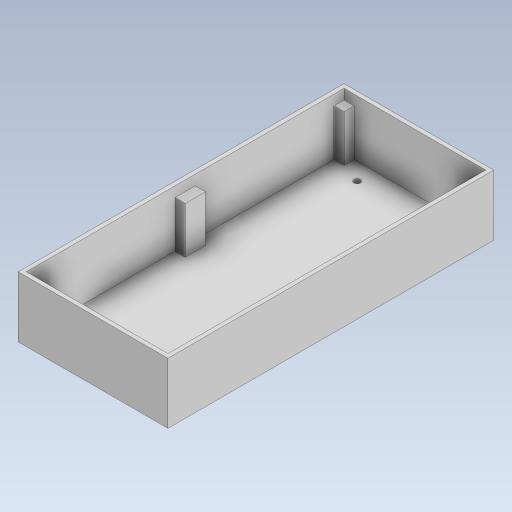
# Autodesk Inventor part: Mounting Master
Saved by Autodesk Inventor 2023.5 (Build 275446000, 446)
## iProperties
Created: 2025-10-29
Part Number: Mounting Master
Material: Generic
Document SubType Name: Modeling
Designer: Guntur
Density: 1 g/cm^3
Appearance: Default
Author: Guntur
## iProperties of the stored document Mounting Master_3DPrint.ipt
Created: 2025-10-29
Part Number: Mounting Master_3DPrint
Material: Generic
Document SubType Name: Modeling
Designer: Guntur
Density: 1 g/cm^3
Appearance: Default
Author: Guntur
Autodesk Inventor part; units mm, degrees
ref_plane "YZ Plane" through (0, 0, 0) normal (1, 0, 0) x (0, 1, 0)
ref_plane "XZ Plane" through (0, 0, 0) normal (0, 1, 0) x (-1, 0, 0)
ref_plane "XY Plane" through (0, 0, 0) normal (0, 0, 1) x (1, 0, 0)
sketch "Sketch1" plane through (0, 0, 0) normal (0, 1, 0) x (-1, 0, 0)
  line L0 (55, 0) -> (-69, 0) construction
  line L1 (0, 72) -> (0, -101) construction
  line L2 (35, 78.5) -> (-35, 78.5)
  line L3 (-35, 78.5) -> (-35, -78.5)
  line L4 (-35, -78.5) -> (35, -78.5)
  line L5 (35, -78.5) -> (35, 78.5)
  line L6 (35, 78.5) -> (-35, -78.5) construction
  line L7 (-35, 78.5) -> (35, -78.5) construction
  line L8 (37, 80.5) -> (-37, 80.5)
  line L9 (-37, 80.5) -> (-37, -80.5)
  line L10 (-37, -80.5) -> (37, -80.5)
  line L11 (37, -80.5) -> (37, 80.5)
  line L12 (37, 80.5) -> (-37, -80.5) construction
  line L13 (-37, 80.5) -> (37, -80.5) construction
  circle A0 centre (20, -70) radius 1.6
  circle A1 centre (20, -70) radius 2.75
  circle A2 centre (-14, -70) radius 1.6
  circle A3 centre (-14, -70) radius 2.75
  circle A4 centre (20, 70) radius 1.6
  circle A5 centre (20, 70) radius 2.75
  circle A6 centre (-14, 70) radius 1.6
  circle A7 centre (-14, 70) radius 2.75
  line L14 (35, 78.5) -> (30, 78.5)
  line L15 (30, 78.5) -> (30, 73.5)
  line L16 (30, 73.5) -> (35, 73.5)
  line L17 (35, 73.5) -> (35, 78.5)
  line L18 (-35, 78.5) -> (-30, 78.5)
  line L19 (-30, 78.5) -> (-30, 73.5)
  line L20 (-30, 73.5) -> (-35, 73.5)
  line L21 (-35, 73.5) -> (-35, 78.5)
  line L22 (35, -78.5) -> (30, -78.5)
  line L23 (30, -78.5) -> (30, -73.5)
  line L24 (30, -73.5) -> (35, -73.5)
  line L25 (35, -73.5) -> (35, -78.5)
  line L26 (-35, -78.5) -> (-30, -78.5)
  line L27 (-30, -78.5) -> (-30, -73.5)
  line L28 (-30, -73.5) -> (-35, -73.5)
  line L29 (-35, -73.5) -> (-35, -78.5)
  line L30 (40, -5) -> (30, -5)
  line L31 (30, -5) -> (30, 5)
  line L32 (30, 5) -> (40, 5)
  line L33 (40, 5) -> (40, -5)
  line L34 (40, -5) -> (30, 5) construction
  line L35 (30, -5) -> (40, 5) construction
  line L36 (-30, -5) -> (-40, -5)
  line L37 (-40, -5) -> (-40, 5)
  line L38 (-40, 5) -> (-30, 5)
  line L39 (-30, 5) -> (-30, -5)
  line L40 (-30, -5) -> (-40, 5) construction
  line L41 (-40, -5) -> (-30, 5) construction
  point P0 (0, 0)
  point P1 (35, 0)
  point P2 (-35, 0)
  point P3 (-35, 5)
  point P4 (-35, -5)
  point P5 (35, -5)
  point P6 (35, 5)
  dimension "d0" = 70
  dimension "d1" = 157
  dimension "d2" = 74
  dimension "d3" = 161
  dimension "d4" = 3.2
  dimension "d5" = 17
  dimension "d6" = 70
  dimension "d7" = 5.5
  dimension "d8" = 3.2
  dimension "d9" = 5.5
  dimension "d10" = 34
  dimension "d11" = 5
  dimension "d12" = 5
  dimension "d13" = 5
  dimension "d14" = 5
  dimension "d15" = 5
  dimension "d16" = 5
  dimension "d17" = 5
  constraints: 84 end point, 16 parallel, 10 horizontal, 10 midpoint, 8 centre point, 8 perpendicular, 4 coincident, 4 symmetric about line, 2 vertical, 5 other
  measures "d0" distance of L4.end L3.end
  measures "d1" distance of L3.end L2.end
  measures "d2" distance of L10.end L9.end
  measures "d3" distance of L9.end L8.end
  measures "d4" diameter of A0
  measures "d5" distance from line of L11 A0.centre
  measures "d6" distance from line of L0 A0.centre
  measures "d7" diameter of A1
  measures "d8" diameter of A2
  measures "d9" diameter of A3
  measures "d10" distance of A2.centre A1.centre
  measures "d11" distance of L15.end L14.end
  measures "d12" distance of L19.end L20.end
  measures "d13" distance of L18.end L19.end
  measures "d14" distance of L23.end L24.end
  measures "d15" distance of L22.end L23.end
  measures "d16" distance of L28.end L27.end
  measures "d17" distance of L27.end L26.end
extrude "Extrusion1" add sketch "Sketch1" along normal blind 2 contours L15 L16 L5 L32 L31 L30 L24 L23 L4 L27 L28 L3 L36 L39 L38 L20 L19 L2 | L5 L30 L31 L32 | L38 L39 L36 L3 | A1 | A3 | A5 | A7
extrude "Extrusion2" add sketch "Sketch1" along normal blind 25 contours L5 L16 L15 L2 | L19 L20 L3 L2 | L5 L30 L31 L32 | L5 L4 L23 L24 | L38 L39 L36 L3 | L28 L27 L4 L3
extrude "Extrusion3" add sketch "Sketch1" along normal blind 30 contours L2 L3 L38 L9 L8 L11 L32 L5 | L32 L11 L30 L5 | L30 L11 L10 L9 L36 L3 L4 L5 | L3 L36 L9 L38
body "Solid1"
